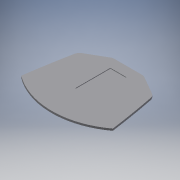
# Autodesk Inventor part: Handle bars holder plates
Saved by Autodesk Inventor 2018 (Build 220112000, 112)
## iProperties
Created: 2018-08-14
Part Number: Handle bars holder plates
Material: Generic
Document SubType Name: Modeling
Designer: ruben
Density: 1 g/cm^3
Sheet Metal Rule: Default_mm
Appearance: Default
Author: ruben
Autodesk Inventor part; units mm, degrees
ref_plane "YZ Plane" through (0, 0, 0) normal (1, 0, 0) x (0, 1, 0)
ref_plane "XZ Plane" through (0, 0, 0) normal (0, 1, 0) x (-1, 0, 0)
ref_plane "XY Plane" through (0, 0, 0) normal (0, 0, 1) x (1, 0, 0)
sketch "Sketch3" plane through (0, 0, 0) normal (0, 0, 1) x (1, 0, 0)
  line L0 (-124.5182, 0) -> (335.753, 0) projected
  line L1 (0, -1648.3682) -> (0, 1648.3682) projected
  line L2 (-58.7652, -57.1704) -> (105.7311, -56.7534) construction
  line L3 (17.7382, 55.0824) -> (1.3397, 26.6795)
  line L4 (17.7382, -55.0824) -> (1.3397, -26.6795)
  line L5 (20, -59) -> (52.7968, -59) construction
  arc A0 (23.8789, 59.7598) -> (17.7382, 55.0824) centre (26.3984, 50.0824) ccw
  arc A1 (17.7382, -55.0824) -> (23.8789, -59.7598) centre (26.3984, -50.0824) ccw
  line L6 (0, 21.6795) -> (0, -21.6795)
  arc A2 (96.0371, -71.9505) -> (96.0371, 71.9505) centre (0, 0) ccw
  line L7 (96.0371, 71.9505) -> (96.0371, -71.9505) construction
  arc A3 (96.0371, 71.9505) -> (23.8789, 59.7598) centre (270, -1177.4058) ccw
  arc A4 (23.8789, -59.7598) -> (96.0371, -71.9505) centre (270, 1177.4058) ccw
  arc A5 (1.3397, 26.6795) -> (0, 21.6795) centre (10, 21.6795) ccw
  arc A6 (0, -21.6795) -> (1.3397, -26.6795) centre (10, -21.6795) ccw
  point P0 (0, 24.359)
  point P1 (0, -24.359)
  point P2 (0, -24.359)
  dimension "d8" = 40
  dimension "d9" = 120
  dimension "d10" = 10
  dimension "d11" = 10
  dimension "d13" = 120
  dimension "d15" = 48.718
  dimension "d16" = 30.7234
  dimension "d17" = 30.7234
  dimension "d18" = 100.1648
  dimension "d19" = 270
  dimension "d20" = 1261.4097
  dimension "d21" = 10
  dimension "d24" = 143.901
  constraints: 15 point on circle, 12 end point, 7 centre point, 6 point on line, 6 tangent, 2 midpoint, 2 symmetric about line, 1 equal length, 1 equal radius, 1 horizontal, 1 parallel, 1 vertical, 1 other
  measures "d8" distance of L5.start point (0, -24.359)
  measures "d9" angle of L5 L4
  measures "d10" radius of A0
  measures "d11" radius of A1
  measures "d13" radius of A2
  measures "d15" distance of point (0, 24.359) point (0, -24.359)
  measures "d16" vertical distance of L3.start point (0, 24.359)
  measures "d17" vertical distance of L4.start point (0, -24.359)
  measures "d18" distance of A0.centre A1.centre
  measures "d19" horizontal distance of A2.centre A3.centre
  measures "d20" radius of A3
  measures "d21" radius of A5
  measures "d24" distance of L7.end L7.start
extrude "Extrusion1" add sketch "Sketch3" along normal blind 3
sketch "Sketch4" plane through (0, 0, 3) normal (0, 0, 1) x (1, 0, 0)
  line L0 (15.466, -12.5) -> (70.466, -12.5)
  line L1 (70.466, -12.5) -> (70.466, 12.5)
  line L2 (70.466, 12.5) -> (15.466, 12.5)
  line L3 (15.466, 12.5) -> (15.466, -12.5)
  line L4 (15.466, -12.5) -> (70.466, 12.5) construction
  line L5 (70.466, -12.5) -> (15.466, 12.5) construction
  point P0 (0, 0)
  point P1 (42.966, 0)
  dimension "d31" = 55
  dimension "d32" = 25
  constraints: 12 end point, 2 midpoint, 2 parallel, 1 horizontal, 1 perpendicular
  measures "d31" distance of L2.end L1.end
  measures "d32" distance of L1.end L0.end
extrude "Extrusion2" cut sketch "Sketch4" against normal blind 1
equation "\"d8\" = d6"
equation "\"d9\" = d7"
equation "\"d11\" = d10"
equation "\"d17\" = d16"
equation "\"BendRadius\" = Thickness"
equation "\"BendReliefWidth\" = Thickness"
equation "\"BendReliefDepth\" = 0.5 * Thickness"
equation "\"CornerReliefSize\" = 4 * Thickness"
equation "\"MinimumRemnant\" = 2 * Thickness"
equation "\"TransitionRadius\" = BendRadius"
equation "\"JacobiRadiusSize\" = BendRadius"
equation "\"GapSize\" = Thickness"
equation "\"d7\" = 120deg"
equation "\"Thickness\" = 0.5"
equation "\"d6\" = 40"
body "Solid1"
